Autodesk Fusion 360 part; units mm, degrees
(part 5 of 5)
  spline S33 degree 5 poles (-128.9509, -52.0549) (-128.953, -52.0614) (-128.9574, -52.0742) (-128.9646, -52.0933) (-128.975, -52.1183) (-128.9895, -52.1491) (-129.005, -52.1794) (-129.021, -52.2096) (-129.0374, -52.2396) (-129.0541, -52.2696) (-129.0709, -52.2995) (-129.0881, -52.3292) (-129.1057, -52.3588) (-129.1237, -52.3882) (-129.1422, -52.4175) (-129.1612, -52.4465) (-129.1805, -52.4753) (-129.2001, -52.5041) (-129.22, -52.5327) (-129.2402, -52.5612) (-129.2607, -52.5895) (-129.2814, -52.6178) (-129.3023, -52.6459) (-129.3236, -52.6739) (-129.3452, -52.7018) (-129.367, -52.7295) (-129.3891, -52.7571) (-129.4115, -52.7846) (-129.4341, -52.812) (-129.457, -52.8392) (-129.48, -52.8664) (-129.5033, -52.8934) (-129.5269, -52.9203) (-129.5506, -52.9471) (-129.5746, -52.9737) (-129.5989, -53.0003) (-129.6233, -53.0267) (-129.648, -53.053) (-129.6728, -53.0792) (-129.6979, -53.1053) (-129.7232, -53.1313) (-129.7487, -53.1572) (-129.7744, -53.1829) (-129.8003, -53.2086) (-129.8264, -53.2341) (-129.8527, -53.2595) (-129.8792, -53.2848) (-129.9058, -53.31) (-129.9327, -53.3351) (-129.9598, -53.36) (-129.987, -53.3849) (-130.0144, -53.4096) (-130.0421, -53.4342) (-130.0699, -53.4588) (-130.0978, -53.4832) (-130.126, -53.5074) (-130.1543, -53.5316) (-130.1828, -53.5557) (-130.2115, -53.5796) (-130.2404, -53.6035) (-130.2694, -53.6272) (-130.2986, -53.6508) (-130.3279, -53.6743) (-130.3575, -53.6977) (-130.3872, -53.721) (-130.417, -53.7442) (-130.447, -53.7672) (-130.4772, -53.7901) (-130.5076, -53.813) (-130.5381, -53.8357) (-130.5687, -53.8583) (-130.5934, -53.8763) (-130.612, -53.8897) (-130.6244, -53.8986) (-130.6306, -53.9031) knots 0 0 0 0 0 0 0.01428571 0.02857143 0.04285714 0.05714286 0.07142857 0.08571429 0.1 0.11428571 0.12857143 0.14285714 0.15714286 0.17142857 0.18571429 0.2 0.21428571 0.22857143 0.24285714 0.25714286 0.27142857 0.28571429 0.3 0.31428571 0.32857143 0.34285714 0.35714286 0.37142857 0.38571429 0.4 0.41428571 0.42857143 0.44285714 0.45714286 0.47142857 0.48571429 0.5 0.51428571 0.52857143 0.54285714 0.55714286 0.57142857 0.58571429 0.6 0.61428571 0.62857143 0.64285714 0.65714286 0.67142857 0.68571429 0.7 0.71428571 0.72857143 0.74285714 0.75714286 0.77142857 0.78571429 0.8 0.81428571 0.82857143 0.84285714 0.85714286 0.87142857 0.88571429 0.9 0.91428571 0.92857143 0.94285714 0.95714286 0.97142857 0.98571429 1 1 1 1 1 1
  line L33 (-128.9509, -52.0549) -> (-128.8165, -51.6448)
  arc A66 (-128.2052, -51.3195) -> (-128.8165, -51.6448) centre (-128.3414, -51.8006) ccw
  arc A67 (-128.2052, -51.3195) -> (-127.4203, -51.5128) centre (-125, -40) ccw
  arc A68 (-127.0301, -52.085) -> (-127.4203, -51.5128) centre (-127.5232, -52.0021) ccw
  line L34 (-127.0301, -52.085) -> (-127.1016, -52.5106)
  spline S34 degree 5 poles (-127.1016, -52.5106) (-127.1027, -52.5173) (-127.1048, -52.5307) (-127.1073, -52.5509) (-127.1097, -52.5779) (-127.1111, -52.6119) (-127.1116, -52.6459) (-127.1113, -52.6801) (-127.1108, -52.7143) (-127.11, -52.7486) (-127.1089, -52.7829) (-127.1076, -52.8172) (-127.1057, -52.8516) (-127.1034, -52.886) (-127.1006, -52.9205) (-127.0973, -52.955) (-127.0936, -52.9895) (-127.0896, -53.0241) (-127.0852, -53.0587) (-127.0806, -53.0933) (-127.0757, -53.1279) (-127.0705, -53.1625) (-127.0649, -53.1972) (-127.0591, -53.2319) (-127.0529, -53.2666) (-127.0465, -53.3013) (-127.0397, -53.336) (-127.0327, -53.3707) (-127.0254, -53.4054) (-127.0178, -53.4402) (-127.01, -53.4749) (-127.0019, -53.5097) (-126.9936, -53.5444) (-126.985, -53.5792) (-126.9761, -53.614) (-126.967, -53.6487) (-126.9576, -53.6835) (-126.948, -53.7183) (-126.9382, -53.753) (-126.9281, -53.7878) (-126.9178, -53.8225) (-126.9072, -53.8573) (-126.8964, -53.892) (-126.8854, -53.9267) (-126.8741, -53.9615) (-126.8627, -53.9962) (-126.8509, -54.0309) (-126.839, -54.0656) (-126.8269, -54.1003) (-126.8145, -54.135) (-126.8019, -54.1696) (-126.7891, -54.2043) (-126.7761, -54.2389) (-126.7629, -54.2735) (-126.7494, -54.3081) (-126.7358, -54.3427) (-126.7219, -54.3773) (-126.7079, -54.4118) (-126.6936, -54.4464) (-126.6791, -54.4809) (-126.6644, -54.5154) (-126.6496, -54.5499) (-126.6345, -54.5843) (-126.6192, -54.6188) (-126.6037, -54.6532) (-126.588, -54.6875) (-126.5722, -54.7219) (-126.5561, -54.7562) (-126.5398, -54.7906) (-126.5234, -54.8248) (-126.5067, -54.8591) (-126.4932, -54.8865) (-126.483, -54.907) (-126.4762, -54.9207) (-126.4728, -54.9275) knots 0 0 0 0 0 0 0.01428571 0.02857143 0.04285714 0.05714286 0.07142857 0.08571429 0.1 0.11428571 0.12857143 0.14285714 0.15714286 0.17142857 0.18571429 0.2 0.21428571 0.22857143 0.24285714 0.25714286 0.27142857 0.28571429 0.3 0.31428571 0.32857143 0.34285714 0.35714286 0.37142857 0.38571429 0.4 0.41428571 0.42857143 0.44285714 0.45714286 0.47142857 0.48571429 0.5 0.51428571 0.52857143 0.54285714 0.55714286 0.57142857 0.58571429 0.6 0.61428571 0.62857143 0.64285714 0.65714286 0.67142857 0.68571429 0.7 0.71428571 0.72857143 0.74285714 0.75714286 0.77142857 0.78571429 0.8 0.81428571 0.82857143 0.84285714 0.85714286 0.87142857 0.88571429 0.9 0.91428571 0.92857143 0.94285714 0.95714286 0.97142857 0.98571429 1 1 1 1 1 1
  arc A69 (-126.4728, -54.9275) -> (-125.5359, -54.9904) centre (-125, -40) ccw
  spline S35 degree 5 poles (-124.5896, -52.6792) (-124.5894, -52.686) (-124.5891, -52.6996) (-124.5893, -52.7199) (-124.5906, -52.747) (-124.5937, -52.7809) (-124.5978, -52.8147) (-124.6026, -52.8485) (-124.6077, -52.8824) (-124.6131, -52.9162) (-124.6187, -52.9501) (-124.6247, -52.9839) (-124.6311, -53.0177) (-124.638, -53.0515) (-124.6454, -53.0853) (-124.6533, -53.1191) (-124.6615, -53.1528) (-124.6702, -53.1865) (-124.6791, -53.2202) (-124.6883, -53.2539) (-124.6978, -53.2875) (-124.7076, -53.3212) (-124.7177, -53.3548) (-124.7281, -53.3884) (-124.7389, -53.4219) (-124.7499, -53.4554) (-124.7613, -53.489) (-124.7729, -53.5224) (-124.7847, -53.5559) (-124.7969, -53.5893) (-124.8093, -53.6227) (-124.8219, -53.656) (-124.8349, -53.6894) (-124.848, -53.7227) (-124.8615, -53.7559) (-124.8751, -53.7892) (-124.8891, -53.8224) (-124.9032, -53.8555) (-124.9177, -53.8887) (-124.9323, -53.9218) (-124.9472, -53.9548) (-124.9623, -53.9879) (-124.9776, -54.0208) (-124.9932, -54.0538) (-125.009, -54.0867) (-125.025, -54.1196) (-125.0412, -54.1524) (-125.0577, -54.1852) (-125.0744, -54.2179) (-125.0913, -54.2507) (-125.1084, -54.2833) (-125.1257, -54.316) (-125.1432, -54.3485) (-125.1609, -54.3811) (-125.1789, -54.4136) (-125.197, -54.446) (-125.2154, -54.4784) (-125.2339, -54.5108) (-125.2527, -54.5431) (-125.2717, -54.5754) (-125.2908, -54.6076) (-125.3102, -54.6398) (-125.3297, -54.6719) (-125.3495, -54.704) (-125.3694, -54.736) (-125.3896, -54.768) (-125.4099, -54.7999) (-125.4304, -54.8318) (-125.4511, -54.8636) (-125.472, -54.8954) (-125.4931, -54.9271) (-125.5101, -54.9525) (-125.523, -54.9715) (-125.5316, -54.9841) (-125.5359, -54.9904) knots 0 0 0 0 0 0 0.01428571 0.02857143 0.04285714 0.05714286 0.07142857 0.08571429 0.1 0.11428571 0.12857143 0.14285714 0.15714286 0.17142857 0.18571429 0.2 0.21428571 0.22857143 0.24285714 0.25714286 0.27142857 0.28571429 0.3 0.31428571 0.32857143 0.34285714 0.35714286 0.37142857 0.38571429 0.4 0.41428571 0.42857143 0.44285714 0.45714286 0.47142857 0.48571429 0.5 0.51428571 0.52857143 0.54285714 0.55714286 0.57142857 0.58571429 0.6 0.61428571 0.62857143 0.64285714 0.65714286 0.67142857 0.68571429 0.7 0.71428571 0.72857143 0.74285714 0.75714286 0.77142857 0.78571429 0.8 0.81428571 0.82857143 0.84285714 0.85714286 0.87142857 0.88571429 0.9 0.91428571 0.92857143 0.94285714 0.95714286 0.97142857 0.98571429 1 1 1 1 1 1
  line L35 (-124.5896, -52.6792) -> (-124.6036, -52.2479)
  arc A70 (-124.1404, -51.7331) -> (-124.6036, -52.2479) centre (-124.1038, -52.2317) ccw
  arc A71 (-124.1404, -51.7331) -> (-123.3367, -51.6463) centre (-125, -40) ccw
  circle A72 centre (-125, -40) radius 4
  line L36 (-120, -40) -> (-120, -37)
  line L37 (-120, -40) -> (-120, -43)
  line L38 (-120, -43) -> (-60, -43)
  line L39 (-60, -43) -> (-60, -37)
  line L40 (-60, -37) -> (-120, -37)
  line L41 (-150, -100) -> (-150, 0)
  line L42 (-180, -43) -> (-240, -43)
  line L43 (-240, -37) -> (-180, -37)
  line L44 (-240, -43) -> (-240, -37)
  line L45 (-180, -40) -> (-180, -43)
  line L46 (-180, -40) -> (-180, -37)
  dimension "d78" = 6
  constraint vertical L36
  constraint parallel L36 L37
  constraint perpendicular L37 L38
  constraint perpendicular L38 L39
  constraint symmetric L36.start L41 L45.start
  constraint symmetric L36.end L41 L43.end
  constraint symmetric L37.end L41 L42.start
  constraint symmetric L38.end L41 L42.end
  constraint symmetric L39.end L41 L43.start
  measures "d78" distance of L38.end L39.end
extrude "Extrude1''''" add sketch "Sketch6" along normal blind 5 separate body contours S7 L7 A14 A15 A16 L8 S8 A17 S9 L9 A18 A19 L36 L37 L38 L40 | S7 L7 A14 A15 A16 L8 S8 A17 S9 L9 A18 A19 L38 L39 L40 makes body 6 in component "BratStanga"
extrude "Extrude1'''''" add sketch "Sketch6" along normal blind 5 separate body contours L42 L43 L44 L45 L46 makes body 7 in component "BratDreapta"
sketch "Sketch7" plane through (0, 9, -8.7312) normal (0, 1, 0) x (-1, 0, 0)
  line L0 (-159.625, -9.7327) -> (-163, -10.9611)
  line L1 (-163, -10.9611) -> (-163, -12.2252)
  line L2 (-163, -12.2252) -> (-159.625, -13.4536)
  line L3 (-159.625, -13.4536) -> (-159.625, -14.4447)
  line L4 (-159.625, -14.4447) -> (-163, -15.6731)
  line L5 (-163, -15.6731) -> (-163, -16.9372)
  line L6 (-163, -16.9372) -> (-159.625, -18.1656)
  line L7 (-159.625, -18.1656) -> (-159.625, -19.1567)
  line L8 (-159.625, -19.1567) -> (-163, -20.3851)
  line L9 (-163, -20.3851) -> (-163, -21.6492)
  line L10 (-163, -21.6492) -> (-159.625, -22.8776)
  line L11 (-159.625, -22.8776) -> (-159.625, -23.8687)
  line L12 (-159.625, -23.8687) -> (-163, -25.0971)
  line L13 (-163, -25.0971) -> (-163, -26.3612)
  line L14 (-163, -26.3612) -> (-159.625, -27.5896)
  line L15 (-159.625, -27.5896) -> (-159.625, -28.5807)
  line L16 (-159.625, -28.5807) -> (-163, -29.8091)
  line L17 (-163, -29.8091) -> (-163, -31.0732)
  line L18 (-163, -31.0732) -> (-159.625, -32.3016)
  line L19 (-159.625, -32.3016) -> (-159.625, -33.2927)
  line L20 (-159.625, -33.2927) -> (-163, -34.5211)
  line L21 (-163, -34.5211) -> (-163, -35.7852)
  line L22 (-163, -35.7852) -> (-159.625, -37.0136)
  line L23 (-159.625, -37.0136) -> (-159.625, -38.0047)
  line L24 (-159.625, -38.0047) -> (-163, -39.2331)
  line L25 (-163, -39.2331) -> (-163, -40.4972)
  line L26 (-163, -40.4972) -> (-159.625, -41.7256)
  line L27 (-159.625, -41.7256) -> (-159.625, -42.7167)
  line L28 (-159.625, -42.7167) -> (-163, -43.9451)
  line L29 (-163, -43.9451) -> (-163, -45.2092)
  line L30 (-163, -45.2092) -> (-159.625, -46.4376)
  line L31 (-159.625, -46.4376) -> (-159.625, -47.4287)
  line L32 (-159.625, -47.4287) -> (-163, -48.6571)
  line L33 (-163, -48.6571) -> (-163, -49.9212)
  line L34 (-163, -49.9212) -> (-159.625, -51.1496)
  line L35 (-159.625, -51.1496) -> (-159.625, -52.1407)
  line L36 (-159.625, -52.1407) -> (-163, -53.3691)
  line L37 (-163, -53.3691) -> (-163, -54.6332)
  line L38 (-163, -54.6332) -> (-159.625, -55.8616)
  line L39 (-159.625, -55.8616) -> (-159.625, -56.8527)
  line L40 (-159.625, -56.8527) -> (-163, -58.0811)
  line L41 (-163, -58.0811) -> (-163, -66.3571)
  line L42 (-163, -66.3571) -> (-137, -66.3571)
  line L43 (-137, -66.3571) -> (-137, -58.0811)
  line L44 (-137, -58.0811) -> (-140.375, -56.8527)
  line L45 (-140.375, -56.8527) -> (-140.375, -55.8616)
  line L46 (-140.375, -55.8616) -> (-137, -54.6332)
  line L47 (-137, -54.6332) -> (-137, -53.3691)
  line L48 (-137, -53.3691) -> (-140.375, -52.1407)
  line L49 (-140.375, -52.1407) -> (-140.375, -51.1496)
  line L50 (-140.375, -51.1496) -> (-137, -49.9212)
  line L51 (-137, -49.9212) -> (-137, -48.6571)
  line L52 (-137, -48.6571) -> (-140.375, -47.4287)
  line L53 (-140.375, -47.4287) -> (-140.375, -46.4376)
  line L54 (-140.375, -46.4376) -> (-137, -45.2092)
  line L55 (-137, -45.2092) -> (-137, -43.9451)
  line L56 (-137, -43.9451) -> (-140.375, -42.7167)
  line L57 (-140.375, -42.7167) -> (-140.375, -41.7256)
  line L58 (-140.375, -41.7256) -> (-137, -40.4972)
  line L59 (-137, -40.4972) -> (-137, -39.2331)
  line L60 (-137, -39.2331) -> (-140.375, -38.0047)
  line L61 (-140.375, -38.0047) -> (-140.375, -37.0136)
  line L62 (-140.375, -37.0136) -> (-137, -35.7852)
  line L63 (-137, -35.7852) -> (-137, -34.5211)
  line L64 (-137, -34.5211) -> (-140.375, -33.2927)
  line L65 (-140.375, -33.2927) -> (-140.375, -32.3016)
  line L66 (-140.375, -32.3016) -> (-137, -31.0732)
  line L67 (-137, -31.0732) -> (-137, -29.8091)
  line L68 (-137, -29.8091) -> (-140.375, -28.5807)
  line L69 (-140.375, -28.5807) -> (-140.375, -27.5896)
  line L70 (-140.375, -27.5896) -> (-137, -26.3612)
  line L71 (-137, -26.3612) -> (-137, -25.0971)
  line L72 (-137, -25.0971) -> (-140.375, -23.8687)
  line L73 (-140.375, -23.8687) -> (-140.375, -22.8776)
  line L74 (-140.375, -22.8776) -> (-137, -21.6492)
  line L75 (-137, -21.6492) -> (-137, -20.3851)
  line L76 (-137, -20.3851) -> (-140.375, -19.1567)
  line L77 (-140.375, -19.1567) -> (-140.375, -18.1656)
  line L78 (-140.375, -18.1656) -> (-137, -16.9372)
  line L79 (-137, -16.9372) -> (-137, -15.6731)
  line L80 (-137, -15.6731) -> (-140.375, -14.4447)
  line L81 (-140.375, -14.4447) -> (-140.375, -13.4536)
  line L82 (-140.375, -13.4536) -> (-137, -12.2252)
  line L83 (-137, -12.2252) -> (-137, -10.9611)
  line L84 (-137, -10.9611) -> (-140.375, -9.7327)
  line L85 (-140.375, -9.7327) -> (-140.375, -8.7416)
  line L86 (-140.375, -8.7416) -> (-137, -7.5132)
  line L87 (-137, -7.5132) -> (-137, -6.3571)
  line L88 (-137, -6.3571) -> (-163, -6.3571)
  line L89 (-163, -6.3571) -> (-163, -7.5132)
  line L90 (-163, -7.5132) -> (-159.625, -8.7416)
  line L91 (-159.625, -8.7416) -> (-159.625, -9.7327)
  line L92 (-137, -6.3571) -> (-163, -6.3571)
  line L93 (-163, -6.3571) -> (-163, -9.3571)
  line L94 (-163, -9.3571) -> (-137, -9.3571)
  line L95 (-137, -9.3571) -> (-137, -6.3571)
  dimension "d83" = 3
  constraint coincident L87.end L88.start
  constraint coincident L88.end L89.start
  constraint perpendicular L92 L93
  constraint perpendicular L85 L94
  measures "d83" distance of L88.end L93.end
extrude "Extrude4'" add sketch "Sketch7" along normal blind 23 contours L90 L91 L93 L94 | L85 L86 L87 L88 L89 L90 L91 L92 L93 L94 L95 | L85 L86 L94 L95 sketch seen with x (1, 0, 0) y (0, 1, 0) z (0, 0, 1) at (0, 0, 5.0883) bodies 3 in component "CompCremaliera"
sketch "Sketch8" plane through (0, 0, -18.0883) normal (0, 0, -1) x (-1, 0, 0)
  line L0 (-163, 9) -> (-159.625, 9)
  line L1 (-159.625, 9) -> (-140.375, 9)
  line L2 (-140.375, 9) -> (-137, 9)
  line L3 (-137, 9) -> (-137, 32)
  line L4 (-137, 32) -> (-163, 32)
  line L5 (-163, 32) -> (-163, 9)
  line L6 (-137, 32) -> (-163, 32)
  line L7 (-163, 32) -> (-163, 29)
  line L8 (-163, 29) -> (-137, 29)
  line L9 (-137, 29) -> (-137, 32)
  constraint coincident L3.end L4.start
  constraint coincident L4.end L5.start
  constraint coincident L5 L7.end
  constraint coincident L3 L8.end
  constraint perpendicular L3 L8
extrude "Extrude5" add sketch "Sketch8" along normal blind 3 contours L3 L4 L5 L6 L7 L8 L9 sketch seen with x (1, 0, 0) y (0, 1, 0) z (0, 0, 1) at (0, 0, 5.0883) bodies 3 in component "CompCremaliera"
sketch "Sketch9" plane through (8.443, 15, 20.328) normal (0, 1, 0) x (-0.985936, 0, 0.167125)
  line L0 (-119.5689, -37.8778) -> (-120.5717, -43.7934)
  line L1 (-120.5717, -43.7934) -> (-61.4155, -53.8209)
  line L2 (-61.4155, -53.8209) -> (-60.4128, -47.9053)
  line L3 (-60.4128, -47.9053) -> (-119.5689, -37.8778)
sketch "Sketch10" plane through (0, 15, 0) normal (0, 1, 0) x (-1, 0, 0)
  line L0 (-120, -37) -> (-120, -43)
  line L1 (-120, -43) -> (-60, -43)
  line L2 (-60, -43) -> (-60, -37)
  line L3 (-60, -37) -> (-120, -37)
  circle A0 centre (-63, -40) radius 2
  circle A1 centre (-63, -40) radius 4
  line L4 (-150, -100) -> (-150, 0)
  circle A2 centre (-237, -40) radius 4
  circle A3 centre (-237, -40) radius 2
  constraint concentric A0 A1
  constraint symmetric A0 L4 A3
  constraint symmetric A1 L4 A2
extrude "Extrude2'''" add sketch "Sketch10" along normal blind 15 contours A0 bodies 6 in component "BratStanga"
extrude "Extrude3'''" add sketch "Sketch10" along normal blind 2 from surface at 15 contours L3 A1 | L1 L2 L3 A1 | L1 A1 | L2 A1 | A0 bodies 6 in component "BratStanga"
extrude "Extrude2''''" add sketch "Sketch10" along normal blind 15 contours A3 bodies 7 in component "BratDreapta"
extrude "Extrude3''''" add sketch "Sketch10" along normal blind 2 from surface at 15 contours A2 | A3 bodies 7 in component "BratDreapta"
copy_body "Body->Comp2" bodies 5 removing the originals makes body 8 in component "CompTel"
sketch "Sketch11" plane through (0, 8, 0) normal (0, 1, 0) x (-1, 0, 0)
  line L0 (-163.7, -105) -> (-163.7, -100)
  line L1 (-163.7, -100) -> (-200, -100)
  line L2 (-200, -100) -> (-200, 0)
  line L3 (-200, 0) -> (-100, 0)
  line L4 (-100, 0) -> (-100, -100)
  line L5 (-100, -100) -> (-136.3, -100)
  line L6 (-136.3, -100) -> (-136.3, -105)
  line L7 (-136.3, -105) -> (-95, -105)
  line L8 (-95, -105) -> (-95, 5)
  line L9 (-95, 5) -> (-205, 5)
  line L10 (-205, 5) -> (-205, -105)
  line L11 (-205, -105) -> (-163.7, -105)
  line L12 (-150, 5) -> (-165, 5)
  line L13 (-150, 5) -> (-135, 5)
  line L14 (-135, 5) -> (-135, 0)
  line L15 (-135, 0) -> (-165, 0)
  line L16 (-165, 0) -> (-165, 5)
  dimension "d112" = 15
  constraint midpoint L9 L12.start
  constraint coincident L9 L12.end
  constraint parallel L9 L13
  constraint coincident L3 L14.end
  constraint perpendicular L3 L14
  constraint coincident L3 L15.end
  constraint perpendicular L12 L16
  measures "d112" distance of L12.start L13.end
extrude "Extrude4''" cut sketch "Sketch11" against normal blind 4 contours L3 L9 L12 L13 L14 L15 L16 bodies 4 in component "compPlaca"
sketch "Sketch12" plane through (0, 4, 0) normal (0, 1, 0) x (-1, 0, 0)
  line L0 (-136.3, -59.5) -> (-136.3, -100)
  line L1 (-136.3, -100) -> (-100, -100)
  line L2 (-100, -100) -> (-100, 0)
  line L3 (-100, 0) -> (-135, 0)
  line L4 (-135, 0) -> (-135, 5)
  line L5 (-135, 5) -> (-147.5, 5)
  line L6 (-147.5, 5) -> (-147.5, -59.5)
  line L7 (-147.5, -59.5) -> (-136.3, -59.5)
  circle A0 centre (-125, -40) radius 3
  circle A1 centre (-130, -80) radius 2
  circle A2 centre (-130, -80) radius 3
  line L8 (-150, -100) -> (-150, 0)
  circle A3 centre (-170, -80) radius 3
  circle A4 centre (-170, -80) radius 2
  dimension "d115" = 4
  dimension "d116" = 6
  constraint concentric A1 A2
  constraint symmetric A1 L8 A4
  constraint symmetric A2 L8 A3
  measures "d115" diameter of A1
  measures "d116" diameter of A2
extrude "Extrude5'" add sketch "Sketch12" along normal blind 4 contours A1 | A4 bodies 4 in component "compPlaca"
extrude "Extrude6" add sketch "Sketch12" along normal blind 2 from surface at 4 contours A1 | A2 | A3 | A4 bodies 4 in component "compPlaca"
sketch "Sketch13" plane through (0, 9, -8.7312) normal (0, 1, 0) x (-1, 0, 0)
  line L0 (-148, -65) -> (-152, -65)
  line L1 (-152, -65) -> (-152, -68)
  line L2 (-152, -68) -> (-148, -68)
  line L3 (-148, -68) -> (-148, -65)
  line L4 (-148, -67) -> (-152, -67)
  constraint horizontal L0
  constraint perpendicular L0 L1
  constraint perpendicular L1 L2
  constraint perpendicular L0 L3
  constraint coincident L3 L4.start
  constraint perpendicular L3 L4
extrude "Extrude6'" add sketch "Sketch13" against normal blind 2.5 contours L0 L1 L3 L4 sketch seen with x (1, 0, 0) y (0, 1, 0) z (0, 0, 1) at (0, 0, 4.9821) bodies 3 in component "CompCremaliera"
extrude "Extrude7" add sketch "Sketch13" against normal blind 7 contours L1 L2 L3 L4 sketch seen with x (1, 0, 0) y (0, 1, 0) z (0, 0, 1) at (0, 0, 4.9821) bodies 3 in component "CompCremaliera"
sketch "Sketch14" plane through (0, 0, 0) normal (1, 0, 0) x (0, 0, -1)
sketch "Sketch15" plane through (214.8294, 0, 0) normal (1, 0, 0) x (0, 0, -1)
  line L0 (6.9805, 19) -> (156.9805, 19)
  line L1 (156.9805, 19) -> (156.9805, 29)
  line L2 (156.9805, 29) -> (6.9805, 29)
  line L3 (6.9805, 29) -> (6.9805, 19)
  line L4 (150, 195) -> (150, 160)
  line L5 (140, 150) -> (60, 150)
  line L6 (50, 160) -> (50, 195)
  line L7 (155, 200) -> (166.2, 200)
  line L8 (170, 196.2) -> (170, 150)
  line L9 (150, 130) -> (50, 130)
  line L10 (30, 150) -> (30, 196.2)
  line L11 (45, 200) -> (33.8, 200)
  arc A0 (150, 130) -> (170, 150) centre (150, 150) ccw
  arc A1 (30, 150) -> (50, 130) centre (50, 150) ccw
  arc A2 (155, 200) -> (150, 195) centre (155, 195) ccw
  arc A3 (50, 195) -> (45, 200) centre (45, 195) ccw
  arc A4 (33.8, 200) -> (30, 196.2) centre (33.8, 196.2) ccw
  arc A5 (170, 196.2) -> (166.2, 200) centre (166.2, 196.2) ccw
  arc A6 (140, 150) -> (150, 160) centre (140, 160) ccw
  arc A7 (50, 160) -> (60, 150) centre (60, 160) ccw
  dimension "d126" = 20
  dimension "d127" = 20
  dimension "d128" = 5
  dimension "d129" = 5
  dimension "d130" = 3.8
  dimension "d131" = 3.8
  dimension "d132" = 10
  dimension "d133" = 10
  constraint vertical L4
  constraint perpendicular L4 L5
  constraint perpendicular L5 L6
  constraint perpendicular L4 L7
  constraint perpendicular L7 L8
  constraint perpendicular L8 L9
  constraint perpendicular L9 L10
  constraint perpendicular L10 L11
  constraint tangent L8 A0
  constraint tangent L9 A0
  constraint tangent L9 A1
  constraint tangent L10 A1
  constraint tangent L7 A2
  constraint tangent L4 A2
  constraint tangent L6 A3
  constraint tangent L11 A3
  constraint tangent L10 A4
  constraint tangent L11 A4
  constraint tangent L8 A5
  constraint tangent L7 A5
  constraint tangent L4 A6
  constraint tangent L5 A6
  constraint tangent L5 A7
  constraint tangent L6 A7
  measures "d126" radius of A0
  measures "d127" radius of A1
  measures "d128" radius of A2
  measures "d129" radius of A3
  measures "d130" radius of A4
  measures "d131" radius of A5
  measures "d132" radius of A6
  measures "d133" radius of A7
extrude "Extrude5''" add sketch "Sketch15" along normal blind 20 separate body contours L4 L5 L6 L7 L8 L9 L10 L11 A0 A1 A2 A3 A4 A5 A6 A7 makes body 9
sketch "Sketch16" plane through (0, 0, -50) normal (0, 0, -1) x (-1, 0, 0)
  line L0 (-214.8294, 160) -> (-214.8294, 195)
  line L1 (-214.8294, 195) -> (-234.8294, 195)
  line L2 (-234.8294, 195) -> (-234.8294, 160)
  line L3 (-234.8294, 160) -> (-214.8294, 160)
  line L4 (-224.8294, 195) -> (-224.8294, 185)
  circle A0 centre (-224.8294, 185) radius 5
  dimension "d136" = 10
  constraint midpoint L1 L4.start
  constraint perpendicular L3 L4
  constraint coincident L4.end A0.centre
  measures "d136" diameter of A0
extrude "Extrude6''" cut sketch "Sketch16" against normal blind 40 contours A0 bodies 9
sketch "Sketch17" plane through (0, 130, 0) normal (0, -1, 0) x (1, 0, 0)
  line L0 (214.8294, -50) -> (214.8294, -150)
  line L1 (214.8294, -150) -> (234.8294, -150)
  line L2 (234.8294, -150) -> (234.8294, -50)
  line L3 (234.8294, -50) -> (214.8294, -50)
move_body "Move1" bodies 9 to x (1, 0, 0) y (0, 1, 0) z (0, 0, 1) at (80, 0, 0)
sketch "Sketch18" plane through (0, 130, 0) normal (0, -1, 0) x (1, 0, 0)
  line L0 (294.8294, -50) -> (294.8294, -150)
  line L1 (294.8294, -150) -> (314.8294, -150)
  line L2 (314.8294, -150) -> (314.8294, -50)
  line L3 (314.8294, -50) -> (294.8294, -50)
  line L4 (330, -150) -> (280, -150)
  line L5 (314.8294, -150) -> (294.8294, -150)
  line L6 (330, -150) -> (330, -70)
  line L7 (330, -70) -> (280, -70)
  line L8 (280, -70) -> (280, -150)
  constraint perpendicular L0 L4
  constraint coincident L1.end L2.start
  constraint coincident L0.end L1.start
  constraint perpendicular L4 L6
  constraint perpendicular L6 L7
  constraint perpendicular L4 L8
extrude "Extrude7'" add sketch "Sketch18" along normal blind 50 contours L0 L1 L2 L4 L5 L7 | L0 L4 L7 L8 | L2 L4 L6 L7 bodies 9
sketch "Sketch19" plane through (0, 0, -150) normal (0, 0, -1) x (-1, 0, 0)
  line L0 (-314.8294, 130) -> (-330, 130)
  line L1 (-330, 130) -> (-330, 80)
  line L2 (-330, 80) -> (-280, 80)
  line L3 (-280, 80) -> (-280, 130)
  line L4 (-280, 130) -> (-294.8294, 130)
  line L5 (-294.8294, 130) -> (-314.8294, 130)
  line L6 (-330, 130) -> (-330, 80)
  line L7 (-280, 80) -> (-280, 130)
  line L8 (-330, 130) -> (-280, 130)
  line L9 (-280, 80) -> (-330, 80)
  line L10 (-289, 84) -> (-321, 84)
  line L11 (-326, 121) -> (-326, 89)
  line L12 (-321, 126) -> (-289, 126)
  line L13 (-284, 89) -> (-284, 121)
  arc A0 (-289, 84) -> (-284, 89) centre (-289, 89) ccw
  arc A1 (-321, 126) -> (-326, 121) centre (-321, 121) ccw
  arc A2 (-284, 121) -> (-289, 126) centre (-289, 121) ccw
  arc A3 (-326, 89) -> (-321, 84) centre (-321, 89) ccw
  dimension "d142" = 5
  dimension "d143" = 5
  dimension "d144" = 5
  dimension "d145" = 5
  constraint coincident L0.end L1.start
  constraint coincident L1.end L2.start
  constraint coincident L2.end L3.start
  constraint coincident L3.end L4.start
  constraint tangent L10 A0
  constraint tangent L13 A0
  constraint tangent L11 A1
  constraint tangent L12 A1
  constraint tangent L13 A2
  constraint tangent L12 A2
  constraint tangent L10 A3
  constraint tangent L11 A3
  measures "d142" radius of A0
  measures "d143" radius of A1
  measures "d144" radius of A2
  measures "d145" radius of A3
extrude "Extrude8" cut sketch "Sketch19" against normal blind 70 contours L10 L11 L12 L13 A0 A1 A2 A3 bodies 9
sketch "Sketch20" plane through (0, 0, 0) normal (0, -1, 0) x (1, 0, 0)
  line L0 (95, -105) -> (205, -105)
  line L1 (205, -105) -> (205, 5)
  line L2 (205, 5) -> (95, 5)
  line L3 (95, 5) -> (95, -105)
  line L4 (175, 5) -> (125, 5)
  line L5 (175, 5) -> (175, -15)
  line L6 (175, -15) -> (125, -15)
  line L7 (125, -15) -> (125, 5)
  constraint coincident L2 L4.start
  constraint coincident L2 L4.end
  constraint perpendicular L4 L5
  constraint perpendicular L5 L6
  constraint perpendicular L4 L7
extrude "Extrude1''''''" add sketch "Sketch20" along normal blind 50 separate body contours L2 L4 L5 L6 L7 makes body 10 in component "prinderePlaca"
sketch "Sketch21" plane through (0, 0, -15) normal (0, 0, -1) x (-1, 0, 0)
  line L0 (-125, 0) -> (-175, 0)
  line L1 (-175, 0) -> (-175, -50)
  line L2 (-175, -50) -> (-125, -50)
  line L3 (-125, -50) -> (-125, 0)
  line L4 (-134, -46) -> (-166, -46)
  line L5 (-171, -41) -> (-171, -9)
  line L6 (-166, -4) -> (-134, -4)
  line L7 (-129, -9) -> (-129, -41)
  line L8 (-129, -46) -> (-171, -4) construction
  line L9 (-171, -46) -> (-129, -4) construction
  arc A0 (-166, -4) -> (-171, -9) centre (-166, -9) ccw
  arc A1 (-134, -46) -> (-129, -41) centre (-134, -41) ccw
  arc A2 (-171, -41) -> (-166, -46) centre (-166, -41) ccw
  arc A3 (-129, -9) -> (-134, -4) centre (-134, -9) ccw
  arc A4 (-130, -9) -> (-134, -5) centre (-134, -9) ccw
  line L10 (-166, -5) -> (-134, -5)
  arc A5 (-166, -5) -> (-170, -9) centre (-166, -9) ccw
  line L11 (-170, -41) -> (-170, -9)
  arc A6 (-170, -41) -> (-166, -45) centre (-166, -41) ccw
  line L12 (-134, -45) -> (-166, -45)
  arc A7 (-134, -45) -> (-130, -41) centre (-134, -41) ccw
  line L13 (-130, -9) -> (-130, -41)
  point P0 (-150, -25)
  dimension "d150" = 42
  dimension "d151" = 42
  dimension "d152" = 5
  dimension "d153" = 5
  dimension "d154" = 5
  dimension "d155" = 5
  dimension "d156" = 1
  constraint horizontal L4
  constraint perpendicular L4 L5
  constraint parallel L4 L6
  constraint parallel L5 L7
  constraint coincident L8 P0
  constraint coincident L9 P0
  constraint coincident L8.end L5
  constraint coincident L8.end L6
  constraint tangent L5 A0
  constraint tangent L6 A0
  constraint coincident L8.start L7
  constraint coincident L8.start L4
  constraint tangent L7 A1
  constraint tangent L4 A1
  constraint coincident L9.start L5
  constraint coincident L9.start L4
  constraint tangent L5 A2
  constraint tangent L4 A2
  constraint coincident L9.end L6
  constraint coincident L9.end L7
  constraint tangent L6 A3
  constraint tangent L7 A3
  measures "d150" distance of L8.end L9.end
  measures "d151" distance of L9.start L8.end
  measures "d152" radius of A0
  measures "d153" radius of A1
  measures "d154" radius of A2
  measures "d155" radius of A3
extrude "Extrude2'''''" add sketch "Sketch21" against normal blind 70 contours A4 L10 A5 L11 A6 L12 A7 L13 bodies 10 in component "prinderePlaca"
sketch "Sketch22" plane through (0, 0, -15) normal (0, 0, -1) x (1, 0, 0)
sketch "Sketch23" plane through (0, 0, -50) normal (0, 0, -1) x (-1, 0, 0)
  circle A0 centre (-304.8294, 185) radius 5
  line L0 (-294.8294, 160) -> (-294.8294, 195)
  line L1 (-294.8294, 195) -> (-314.8294, 195)
  line L2 (-314.8294, 195) -> (-314.8294, 160)
  line L3 (-314.8294, 160) -> (-294.8294, 160)
  circle A1 centre (-375, 185) radius 5
  line L4 (-383, 180.3812) -> (-375, 175.7624)
  line L5 (-375, 175.7624) -> (-367, 180.3812)
  line L6 (-367, 180.3812) -> (-367, 189.6188)
  line L7 (-367, 189.6188) -> (-375, 194.2376)
  line L8 (-375, 194.2376) -> (-383, 189.6188)
  line L9 (-383, 189.6188) -> (-383, 180.3812)
  point P0 (-375, 185)
  dimension "d159" = 10
  dimension "d160" = 8
  constraint coincident P0 A1.centre
  measures "d159" diameter of A1
  measures "d160" distance of P0 L9
extrude "Extrude1'''''''" add sketch "Sketch23" along normal blind 30 separate body contours L4 L5 L6 L7 L8 L9 makes body 11 in component "SurubMenghina"
extrude "Extrude2''''''" add sketch "Sketch23" along normal blind 150 contours A1 bodies 11 in component "SurubMenghina"
copy_body "Body->Comp3" bodies 9 removing the originals makes body 12 in component "Menghina"
thread "Thread1" "ISO Metric Trapezoidal Threads 10.0 TR10x2 TR10x2 7e" major diameter 9.91 minor diameter 7.3455 pitch 2 angle 30 modelled right hand crest width 0.7117 on face at (377.0564, 189.5575, -120) crest through (370.045, 185, -79.5) on bodies 11 in component "SurubMenghina"
thread "Thread1'" "ISO Metric Trapezoidal Threads 10.0 TR10x2 TR10x2 7H" major diameter 10.5 minor diameter 8.118 pitch 2 angle 30 modelled right hand crest width 0.7302 on face at (303.237, 189.7396, -36.6667) crest through (300.7704, 185, -49.5) on bodies 12 in component "Menghina"
sketch "Sketch24" plane through (0, 0, 0) normal (0, 0, 1) x (1, 0, 0)
component "Spur Gear 18 teeth" placed x (0.945428, 0, -0.325832) y (0, 1, 0) z (0.325832, 0, 0.945428) at (19.8548, 0, 38.5461)
component "Spur Gear 18 teeth" placed x (0.945428, 0, 0.325832) y (0, 1, 0) z (-0.325832, 0, 0.945428) at (43.7883, 0, -42.9119)
component "CompCremaliera" placed x (1, 0, 0) y (0, 1, 0) z (0, 0, 1) at (0, 0, 6.0195)
component "compPlaca" placed x (1, 0, 0) y (0, 1, 0) z (0, 0, 1) at (0, 0, 0)
component "BratStanga" placed x (0.680171, 0, 0.733054) y (0, 1, 0) z (-0.733054, 0, 0.680171) at (10.6565, 0, -104.4249)
component "BratDreapta" placed x (0.680171, 0, -0.733054) y (0, 1, 0) z (0.733054, 0, 0.680171) at (85.2923, 0, 115.4912)
component "CompTel" placed x (1, 0, 0) y (0, 1, 0) z (0, 0, 1) at (334.8294, 9, -181.9805)
component "prinderePlaca" placed x (1, 0, 0) y (0, 1, 0) z (0, 0, 1) at (0, 0, 0)
component "SurubMenghina" placed x (-1, 0, 0) y (0, -1, 0) z (0, 0, 1) at (525.1706, 80, 295)
component "Menghina" placed x (-1, 0, 0) y (0, -1, 0) z (0, 0, 1) at (455, 80, 205)
